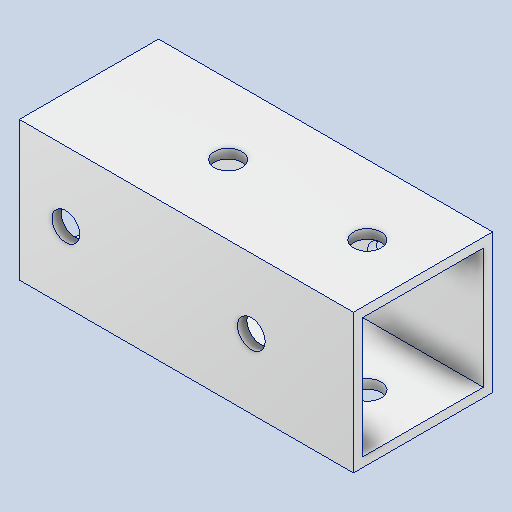
# Autodesk Inventor part: hand-grab-v2-ASP-arm-F-1
Saved by Autodesk Inventor 2025.1 (Build 291241000, 241)
## iProperties
Created: 2024-10-15
Part Number: hand-grab-v2-ASP-arm-F-1
Material: アルミニウム 6061
Document SubType Name: Modeling
Designer: haruy
Density: 2.7 g/cm^3
Appearance: アルミニウム - フラット
Author: haruy
Autodesk Inventor part; units mm, degrees
ref_plane "YZ Plane" through (0, 0, 0) normal (1, 0, 0) x (0, 1, 0)
ref_plane "XZ Plane" through (0, 0, 0) normal (0, 1, 0) x (-1, 0, 0)
ref_plane "XY Plane" through (0, 0, 0) normal (0, 0, 1) x (1, 0, 0)
sketch "スケッチ1" plane through (0, 0, 0) normal (1, 0, 0) x (0, 1, 0)
  line L0 (0, 0) -> (15, 0)
  line L1 (15, 0) -> (15, -15)
  line L2 (15, -15) -> (0, -15)
  line L3 (0, -15) -> (0, 0)
  line L4 (14, -14) -> (14, -1)
  line L5 (14, -1) -> (1, -1)
  line L6 (1, -1) -> (1, -14)
  line L7 (1, -14) -> (14, -14)
  dimension "d0" = 15
  dimension "d1" = 15
  dimension "d2" = 1
  constraints: 16 end point, 4 parallel, 2 perpendicular, 1 horizontal, 3 other
  measures "d0" distance of L1.end L2.end
  measures "d1" distance of L0.end L1.end
  measures "d2" distance between parallel lines of L1 L4
extrude "押し出し1" add sketch "スケッチ1" along normal blind 36
sketch "スケッチ2" plane through (0, 0, 0) normal (0, 0, 1) x (1, 0, 0)
  line L0 (0, 15) -> (0, 0) projected
  line L1 (0, 0) -> (36, 0) projected
  point P0 (5, 7.5)
  point P1 (25, 7.5)
  dimension "d5" = 5
  dimension "d6" = 20
  dimension "d7" = 7.5
  dimension "d8" = 7.5
  measures "d5" distance from line of L0 point (5, 7.5)
  measures "d6" distance of point (25, 7.5) point (5, 7.5)
  measures "d7" distance from line of point (5, 7.5) L1
  measures "d8" distance from line of point (25, 7.5) L1
sketch "スケッチ3" plane through (0, 15, 0) normal (0, 1, 0) x (1, 0, 0)
  line L0 (0, 15) -> (0, 0) projected
  line L1 (0, 0) -> (36, 0) projected
  point P0 (15, 7.5)
  point P1 (30, 7.5)
  dimension "d9" = 15
  dimension "d10" = 15
  dimension "d11" = 7.5
  dimension "d12" = 7.5
  measures "d9" distance from line of point (15, 7.5) L0
  measures "d10" distance of point (30, 7.5) point (15, 7.5)
  measures "d11" distance from line of point (15, 7.5) L1
  measures "d12" distance from line of point (30, 7.5) L1
hole "穴1" at (5, 7.5, 0) at (25, 7.5, 0) direction (0, 0, -1) diameter 3 end through all
hole "穴2" at (15, 15, -7.5) at (30, 15, -7.5) direction (0, -1, 0) diameter 3 end through all
equation "\"d8\" = d7"
equation "\"d12\" = d11"
